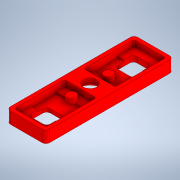
# Autodesk Inventor part: LineSensorPlate
Saved by Autodesk Inventor 2021 (Build 250183000, 183)
## iProperties
Created: 2022-02-28
Part Number: LineSensorPlate
Material: Generic
Document SubType Name: Modeling
Designer: ermoz
Density: 1 g/cm^3
Appearance: Default
Author: ermoz
Autodesk Inventor part; units mm, degrees
ref_plane "YZ Plane" through (0, 0, 0) normal (1, 0, 0) x (0, 1, 0)
ref_plane "XZ Plane" through (0, 0, 0) normal (0, 1, 0) x (-1, 0, 0)
ref_plane "XY Plane" through (0, 0, 0) normal (0, 0, 1) x (1, 0, 0)
sketch "Sketch1" plane through (0, 0, 0) normal (0, 1, 0) x (-1, 0, 0)
  line L0 (0, 0) -> (8, 0)
  line L1 (8, 0) -> (8, -13)
  line L2 (8, -13) -> (0, -13)
  line L3 (0, -13) -> (0, 0)
  line L4 (8.2, -13.2) -> (8.2, 0.2)
  line L5 (8.2, 0.2) -> (-0.2, 0.2)
  line L6 (-0.2, 0.2) -> (-0.2, -13.2)
  line L7 (-0.2, -13.2) -> (8.2, -13.2)
  line L8 (0, -18.4) -> (8, -18.4)
  line L9 (8, -18.4) -> (8, -31.4)
  line L10 (8, -31.4) -> (0, -31.4)
  line L11 (0, -31.4) -> (0, -18.4)
  line L12 (8.2, -31.6) -> (8.2, -18.2)
  line L13 (8.2, -18.2) -> (-0.2, -18.2)
  line L14 (-0.2, -18.2) -> (-0.2, -31.6)
  line L15 (-0.2, -31.6) -> (8.2, -31.6)
  line L16 (9.2, 1.2) -> (-1.2, 1.2)
  line L17 (-1.2, 1.2) -> (-1.2, -32.6)
  line L18 (-1.2, -32.6) -> (9.2, -32.6)
  line L19 (9.2, -32.6) -> (9.2, 1.2)
  circle A0 centre (4, -15.7) radius 1.75
  line L20 (4, -18.2) -> (4, -13.2)
  dimension "d0" = 8
  dimension "d1" = 13
  dimension "d2" = 0.2
  dimension "d3" = 0.2
  dimension "d4" = 3.5
  dimension "d5" = 2.5
  dimension "d6" = 2.5
  dimension "d7" = 1
  dimension "d8" = 1
  dimension "d9" = 1
  dimension "d10" = 1
  constraints: 42 end point, 10 parallel, 5 perpendicular, 3 horizontal, 3 midpoint, 2 equal length, 1 centre point, 1 collinear, 6 other
  measures "d0" distance of L1.end L2.end
  measures "d1" distance of L0.end L1.end
  measures "d2" distance between parallel lines of L1 L4
  measures "d3" distance between parallel lines of L9 L12
  measures "d4" diameter of A0
  measures "d5" distance from line of L7 A0.centre
  measures "d6" distance from line of L13 A0.centre
  measures "d7" distance between parallel lines of L16 L5
  measures "d8" distance between parallel lines of L18 L15
  measures "d9" distance between parallel lines of L19 L12
  measures "d10" distance between parallel lines of L17 L14
extrude "Extrusion1" add sketch "Sketch1" along normal blind 1.6 contours L19 L18 L17 L16
sketch "Sketch2" plane through (0, 0, 0) normal (0, -1, 0) x (1, 0, 0)
  line L0 (-9.2, 1.2) -> (1.2, 1.2) projected
  line L1 (1.2, -32.6) -> (-9.2, -32.6) projected
  line L2 (1.2, 1.2) -> (-9.2, 1.2)
  line L3 (-9.2, 1.2) -> (-9.2, -32.6)
  line L4 (-9.2, -32.6) -> (1.2, -32.6)
  line L5 (1.2, -32.6) -> (1.2, 1.2)
  circle A0 centre (-4, -15.7) radius 1.75 projected
  circle A1 centre (-4, -15.7) radius 1.75
  line L6 (-1.5, -24.7) -> (-6.5, -24.7)
  line L7 (-6.5, -24.7) -> (-6.5, -29.7)
  line L8 (-6.5, -29.7) -> (-1.5, -29.7)
  line L9 (-1.5, -29.7) -> (-1.5, -24.7)
  line L10 (-1.5, -1.7) -> (-6.5, -1.7)
  line L11 (-6.5, -1.7) -> (-6.5, -6.7)
  line L12 (-6.5, -6.7) -> (-1.5, -6.7)
  line L13 (-1.5, -6.7) -> (-1.5, -1.7)
  line L14 (-8.2, -18.2) -> (-8.2, -31.6) projected
  line L15 (-8.2, -31.6) -> (0.2, -31.6) projected
  line L16 (0.2, -18.2) -> (-8.2, -18.2) projected
  line L17 (-4, -18.2) -> (-4, -23.5281)
  line L18 (-8.2, -13.2) -> (0.2, -13.2) projected
  line L19 (0.2, 0.2) -> (-8.2, 0.2) projected
  point P0 (0, 0)
  dimension "d14" = 5
  dimension "d15" = 1.9
  dimension "d16" = 5
  dimension "d39" = 1.9
  constraints: 26 end point, 6 parallel, 3 horizontal, 3 perpendicular, 2 collinear, 1 centre point, 1 coincident, 1 midpoint, 1 point on line, 1 vertical, 1 other
  measures "d14" distance of L6.start L6.end
  measures "d15" distance between parallel lines of L15 L8
  measures "d16" distance of L8.end L6.start
  measures "d39" distance between parallel lines of L19 L10
extrude "Extrusion2" add sketch "Sketch2" along normal blind 1.5
sketch "Sketch3" plane through (0, 0, 0) normal (0, 1, 0) x (1, 0, 0)
  circle A0 centre (-4, 10.8) radius 1.175
  circle A1 centre (-4, 20.6) radius 1.175
  line L0 (0.2, 18.2) -> (-8.2, 18.2) projected
  circle A2 centre (-4, 15.7) radius 1.75 projected
  line L1 (0.2, -0.2) -> (-8.2, -0.2) projected
  line L2 (-6.5, 24.7) -> (-1.5, 24.7) projected
  line L3 (-6.5, 1.7) -> (-1.5, 1.7) projected
  line L4 (-1.5, 6.7) -> (-6.5, 6.7) projected
  point P0 (0, 0)
  dimension "d22" = 2.35
  dimension "d37" = 4.1
  dimension "d40" = 4.1
  constraints: 2 centre point, 2 vertical alignment, 1 equal radius
  measures "d22" diameter of A1
  measures "d37" distance from line of L2 A1.centre
  measures "d40" distance from line of L4 A0.centre
extrude "Extrusion3" add sketch "Sketch3" along normal blind 1.4 contours A0 | A1
chamfer "Chamfer1" distance 2 angle 45 1 edges at (-5.75, -1.5, -15.7)
fillet "Fillet1" radius 1 4 edges at (-9.2, 0.05, 1.2) (1.2, 0.05, 1.2) (-9.2, 0.05, -32.6) (1.2, 0.05, -32.6)
fillet "Fillet2" radius 1 8 edges at (-6.5, -0.75, -1.7) (-1.5, -0.75, -1.7) (-1.5, -0.75, -6.7) (-6.5, -0.75, -6.7) (-6.5, -0.75, -24.7) (-1.5, -0.75, -24.7) (-1.5, -0.75, -29.7) (-6.5, -0.75, -29.7)
fillet "Fillet3" radius 0.5 8 edges at (0.2, 0.8, -31.6) (-8.2, 0.8, -31.6) (-8.2, 0.8, -18.2) (0.2, 0.8, -18.2) (0.2, 0.8, -13.2) (-8.2, 0.8, -13.2) (-8.2, 0.8, 0.2) (0.2, 0.8, 0.2)
sketch "Sketch4" plane through (0, 0, 0) normal (0, 1, 0) x (1, 0, 0)
  line L0 (-8.2, 27.2) -> (0.2, 27.2)
  line L1 (0.2, 27.2) -> (0.2, 20.6)
  line L2 (0.2, 20.6) -> (-8.2, 20.6)
  line L3 (-8.2, 20.6) -> (-8.2, 27.2)
  line L4 (-8.2, 4.2) -> (0.2, 4.2)
  line L5 (0.2, 4.2) -> (0.2, 10.8)
  line L6 (0.2, 10.8) -> (-8.2, 10.8)
  line L7 (-8.2, 10.8) -> (-8.2, 4.2)
  line L8 (-8.2, 18.7) -> (-8.2, 31.1) projected
  line L9 (0.2, 31.1) -> (0.2, 18.7) projected
  line L10 (-5.5, 24.7) -> (-2.5, 24.7) projected
  circle A0 centre (-4, 20.6) radius 1.175 projected
  circle A1 centre (-4, 10.8) radius 1.175 projected
  line L11 (-5.5, 1.7) -> (-2.5, 1.7) projected
  line L12 (-1.5, 25.7) -> (-1.5, 28.7) projected
  line L13 (-1.5, 2.7) -> (-1.5, 5.7) projected
  point P0 (0, 0)
  point P1 (-5.175, 10.8)
  point P2 (-2.825, 10.8)
  point P3 (-5.175, 20.6)
  point P4 (-2.825, 20.6)
  point P5 (-1.5, 27.2)
  point P6 (-1.5, 4.2)
  constraints: 16 end point, 4 collinear, 4 midpoint, 4 parallel, 2 horizontal, 2 perpendicular, 2 point on line
extrude "Extrusion4" cut sketch "Sketch4" against normal blind 0.5 contours L0 L1 L2 A0 L3 | L7 L6 A1 L5 L4 | A1 L6 | L6 A1
equation "\"d3\" = d2"
equation "\"d6\" = d5"
equation "\"d8\" = d7"
equation "\"d10\" = d9"
equation "\"d39\" = d15"
equation "\"d40\" = d37"
body "Solid1"
